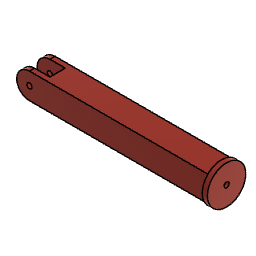
segundobrazo v7 (Autodesk Fusion 360 design; units mm, degrees)
Autodesk Fusion 360 part; units mm, degrees
sketch "Sketch2" plane through (0, 0, 0) normal (0, 1, 0) x (1, 0, 0)
  line L0 (0, -50) -> (700, -50)
  arc A0 (700, -50) -> (700, 50) centre (700, 0) ccw
  line L1 (700, 50) -> (0, 50)
  arc A1 (0, 50) -> (0, -50) centre (0, 0) ccw
  line L2 (0, 0) -> (700, 0) construction
  circle A2 centre (0, 0) radius 10
  line L3 (700, -50) -> (700, 50)
  dimension "d2" = 100
  dimension "d3" = 20
  constraint tangent L0 A0
  constraint tangent A0 L1
  constraint parallel L0 L1
  constraint tangent L1 A1
  constraint tangent L0 A1
  constraint horizontal L2
  constraint coincident A1.centre L2.start
  constraint concentric A1 A2
  measures "d2" diameter of A0
  measures "d3" diameter of A2
extrude "Extrude1" add sketch "Sketch2" along normal blind 100 contours L0 L1 A1 L3
sketch "Sketch3" plane through (0, 0, 50) normal (0, 0, 1) x (-1, 0, 0)
  line L0 (0, 0) -> (-700, 0)
  line L1 (-700, 0) -> (-700, -100)
  line L2 (-700, -100) -> (0, -100)
  line L3 (0, -100) -> (0, 0)
  line L4 (-60, -100) -> (-60, 0)
  line L5 (-60, -80) -> (50, -80)
  line L6 (-60, -20) -> (50, -20)
  line L7 (50, -80) -> (50, -20)
  dimension "d6" = 20
  dimension "d7" = 20
  constraint coincident L2 L4.start
  constraint coincident L0 L4.end
  constraint perpendicular L0 L4
  constraint coincident L4 L5.start
  constraint perpendicular L4 L5
  constraint coincident L4 L6.start
  constraint perpendicular L4 L6
  constraint perpendicular L6 L7
  measures "d6" distance of L2 L5
  measures "d7" distance of L0 L6
extrude "Extrude2" cut sketch "Sketch3" against normal blind 110 contours L3 L5 L6 L7 | L3 L4 L5 L6
sketch "Sketch4" plane through (700, 0, 0) normal (1, 0, 0) x (0, 1, 0)
  line L0 (0, 50) -> (0, -50)
  line L1 (0, -50) -> (100, -50)
  line L2 (100, -50) -> (100, 50)
  line L3 (100, 50) -> (0, 50)
  circle A0 centre (50, 0) radius 75
  dimension "d10" = 150
  measures "d10" diameter of A0
extrude "Extrude3" add sketch "Sketch4" along normal blind 20 contours L0 L1 L2 L3 | A0
sketch "Sketch5" plane through (720, 0, 0) normal (1, 0, 0) x (0, 1, 0)
  circle A0 centre (50, 0) radius 75
  circle A1 centre (50, 0) radius 10
  dimension "d13" = 20
  constraint concentric A0 A1
  measures "d13" diameter of A1
extrude "Extrude4" cut sketch "Sketch5" against normal blind 20 contours A1
scale "Scale1" factor 2.5 about (0, 0, 0) bodies 1
